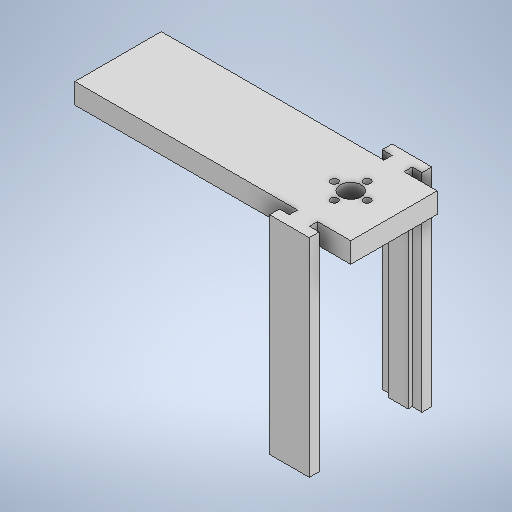
# Autodesk Inventor part: ClawGrip
Saved by Autodesk Inventor 2027 (Build 310192060, 192F)
## iProperties
Created: 2026-06-30
Part Number: ClawGrip
Material: Generic
Document SubType Name: Modeling
Designer: 13129
Density: 1 g/cm^3
Appearance: Default
Author: 13129
Autodesk Inventor part; units mm, degrees
ref_plane "YZ Plane" through (0, 0, 0) normal (1, 0, 0) x (0, 1, 0)
ref_plane "XZ Plane" through (0, 0, 0) normal (0, 1, 0) x (-1, 0, 0)
ref_plane "XY Plane" through (0, 0, 0) normal (0, 0, 1) x (1, 0, 0)
sketch "Sketch1" plane through (0, 0, 0) normal (0, 1, 0) x (-1, 0, 0)
  line L0 (0, 0) -> (42.3, 0)
  line L1 (42.3, 0) -> (42.3, -42.3)
  line L2 (42.3, -42.3) -> (0, -42.3)
  line L3 (0, -42.3) -> (0, 0)
  circle A0 centre (21.15, -21.15) radius 5.15
  circle A1 centre (29.15, -21.15) radius 1.8
  circle A2 centre (21.15, -21.15) radius 8
  circle A3 centre (21.15, -13.15) radius 1.8
  circle A4 centre (13.15, -21.15) radius 1.8
  circle A5 centre (21.15, -29.15) radius 1.8
  point P0 (0, -21.15)
  point P1 (21.15, -42.3)
  dimension "d4" = 16
  dimension "d0" = 42.3
  dimension "d2" = 10.3
  dimension "d3" = 3.6
  dimension "d7" = 360
  constraints: 8 end point, 5 centre point, 4 perpendicular, 3 horizontal alignment, 2 midpoint, 1 coincident, 1 horizontal, 1 vertical alignment, 11 other
  measures "d0" distance of L0.start L0.end
  measures "d2" diameter of A0
  measures "d3" diameter of A1
extrude "Extrusion1" add sketch "Sketch1" along normal blind 10 contours L0 L1 L2 L3 | A1 A2 A5 A4 A3
sketch "Sketch2" plane through (0, 10, 0) normal (0, 1, 0) x (1, 0, 0)
  line L0 (-42.3, 0) -> (0, 0) construction
  circle A0 centre (-13.15, 21.15) radius 1.8 construction
  circle A1 centre (-29.15, 21.15) radius 1.8 construction
  line L1 (-42.3, 0) -> (0, 0) construction
  line L2 (-16.25, 0) -> (-16.25, -3.81)
  line L3 (-16.25, -3.81) -> (-26.05, -3.81)
  line L4 (-26.05, -3.81) -> (-26.05, 0)
  line L5 (-26.05, 0) -> (-16.25, 0)
  line L6 (-13.15, 21.15) -> (-29.15, 21.15)
  line L7 (-42.3, 42.3) -> (0, 42.3) construction
  line L8 (-42.3, 42.3) -> (0, 42.3) construction
  line L9 (-16.25, 42.3) -> (-16.25, 46.11)
  line L10 (-16.25, 46.11) -> (-26.05, 46.11)
  line L11 (-26.05, 46.11) -> (-26.05, 42.3)
  line L12 (-26.05, 42.3) -> (-16.25, 42.3)
  line L13 (-16.25, 46.11) -> (-16.25, 46.31)
  line L14 (-16.25, 46.31) -> (-11.424, 46.31)
  line L15 (-11.424, 46.31) -> (-11.424, 51.136)
  line L16 (-26.05, 46.11) -> (-26.05, 46.31)
  line L17 (-26.05, 46.31) -> (-30.876, 46.31)
  line L18 (-30.876, 46.31) -> (-30.876, 51.136)
  line L19 (-30.876, 51.136) -> (-11.424, 51.136)
  line L20 (-16.25, -3.81) -> (-16.25, -4.01)
  line L21 (-16.25, -4.01) -> (-11.424, -4.01)
  line L22 (-11.424, -4.01) -> (-11.424, -8.836)
  line L23 (-26.05, -3.81) -> (-26.05, -4.01)
  line L24 (-26.05, -4.01) -> (-30.876, -4.01)
  line L25 (-30.876, -4.01) -> (-30.876, -8.836)
  line L26 (-30.876, -8.836) -> (-11.424, -8.836)
  point P0 (-21.15, -3.81)
  point P1 (-21.15, 0)
  point P2 (-21.15, 46.11)
  point P3 (-21.15, 42.3)
  dimension "d11" = 3.81
  dimension "d12" = 9.8
  dimension "d28" = 0.2
  dimension "d29" = 4.826
  dimension "d30" = 4.826
  dimension "d31" = 0.2
  dimension "d32" = 4.826
  dimension "d33" = 4.826
  constraints: 50 end point, 12 symmetric about line, 6 perpendicular, 4 point on line, 2 horizontal, 2 midpoint, 2 vertical, 1 collinear, 1 vertical alignment
  measures "d11" distance of L2.start L2.end
  measures "d12" distance of L2.end L3.end
  measures "d28" distance of L9.end L13.end
  measures "d29" distance of L13.end L14.end
  measures "d30" distance of L14.end L15.end
  measures "d31" distance of L10.end L16.end
  measures "d32" distance of L16.end L17.end
  measures "d33" distance of L17.end L18.end
extrude "Extrusion2" add sketch "Sketch2" against normal blind 10
sketch "Sketch3" plane through (0, 0, 0) normal (0, -1, 0) x (1, 0, 0)
  circle A0 centre (-13.15, -21.15) radius 1.8 construction
  circle A1 centre (-29.15, -21.15) radius 1.8 construction
  line L0 (-13.15, -21.15) -> (-29.15, -21.15)
  line L1 (-16.25, 0) -> (-16.25, 4.01) construction
  line L2 (-11.424, 4.01) -> (-11.424, 8.836) construction
  line L3 (-30.876, 8.836) -> (-30.876, 4.01) construction
  line L4 (-30.876, 4.01) -> (-26.05, 4.01) construction
  line L5 (-26.05, 4.01) -> (-26.05, 0) construction
  line L6 (-16.25, 4.01) -> (-11.424, 4.01)
  line L7 (-11.424, 4.01) -> (-11.424, 8.836)
  line L8 (-11.424, 8.836) -> (-30.876, 8.836)
  line L9 (-30.876, 8.836) -> (-30.876, 4.01)
  line L10 (-30.876, 4.01) -> (-26.05, 4.01)
  line L11 (-26.05, 4.01) -> (-26.05, 2.105)
  line L12 (-26.05, 2.105) -> (-16.25, 2.005)
  line L13 (-16.25, 4.01) -> (-16.25, 2.005)
  line L14 (-16.25, -42.3) -> (-16.25, -46.31) construction
  line L15 (-16.25, -46.31) -> (-11.424, -46.31) construction
  line L16 (-11.424, -46.31) -> (-11.424, -51.136) construction
  line L17 (-11.424, -51.136) -> (-30.876, -51.136) construction
  line L18 (-30.876, -51.136) -> (-30.876, -46.31) construction
  line L19 (-30.876, -46.31) -> (-26.05, -46.31) construction
  line L20 (-26.05, -46.31) -> (-26.05, -42.3) construction
  line L21 (-16.25, -46.31) -> (-11.424, -46.31)
  line L22 (-11.424, -46.31) -> (-11.424, -51.136)
  line L23 (-11.424, -51.136) -> (-30.876, -51.136)
  line L24 (-30.876, -51.136) -> (-30.876, -46.31)
  line L25 (-30.876, -46.31) -> (-26.05, -46.31)
  line L26 (-26.05, -46.31) -> (-26.05, -44.405)
  line L27 (-26.05, -44.405) -> (-16.25, -44.305)
  line L28 (-16.25, -46.31) -> (-16.25, -44.305)
  dimension "d34" = 1.905
  constraints: 48 end point, 6 symmetric about line, 4 collinear, 2 perpendicular, 2 point on line, 1 horizontal, 1 midpoint
  measures "d34" distance of L4.end L11.end
extrude "Extrusion3" add sketch "Sketch3" along normal blind 91.6
sketch "Sketch4" plane through (0, 10, 0) normal (0, 1, 0) x (1, 0, 0)
  line L0 (-42.3, 0) -> (-135.01, 0)
  line L1 (-135.01, 0) -> (-135.01, 42.3)
  line L2 (-135.01, 42.3) -> (-42.3, 42.3)
  line L3 (-42.3, 0) -> (-42.3, 42.3)
  dimension "d17" = 92.71
  constraints: 8 end point, 3 perpendicular, 1 horizontal
  measures "d17" distance of L0.start L0.end
extrude "Extrusion4" add sketch "Sketch4" against normal blind 10
sketch "Sketch5" plane through (0, 0, 0) normal (0, -1, 0) x (1, 0, 0)
  line L0 (-135.01, 0) -> (-135.01, -42.3) construction
  line L1 (-122.31, -36.0725) -> (-51.19, -36.0725)
  line L2 (-51.19, -36.0725) -> (-51.19, -6.2275)
  line L3 (-51.19, -6.2275) -> (-122.31, -6.2275)
  line L4 (-122.31, -6.2275) -> (-122.31, -36.0725)
  point P0 (-135.01, -7.62)
  point P1 (-135.01, -34.68)
  point P2 (-122.31, -21.15)
  point P3 (-135.01, -21.15)
  dimension "d35" = 71.12
  dimension "d36" = 29.845
  dimension "d37" = 12.7
  constraints: 8 end point, 2 midpoint, 2 parallel, 1 horizontal, 1 horizontal alignment, 1 perpendicular
  measures "d35" distance of L3.end L2.end
  measures "d36" distance of L2.end L1.end
  measures "d37" distance between parallel lines of L0 L4
extrude "Extrusion5" cut sketch "Sketch5" against normal blind 5
sketch "Sketch6" plane through (0, 10, 0) normal (0, 1, 0) x (1, 0, 0)
  line L0 (-135.01, 0) -> (-26.05, 0) construction
  line L1 (-30.876, -8.836) -> (-11.424, -8.836) construction
  line L2 (0, 0) -> (0, 42.3) construction
  line L3 (-11.424, 51.136) -> (-30.876, 51.136) construction
  line L4 (-30.876, 51.136) -> (-30.876, 46.31) construction
  line L5 (-26.05, 42.3) -> (-135.01, 42.3) construction
  line L6 (-135.01, 42.3) -> (-135.01, 0) construction
  circle A0 centre (-21.15, 21.15) radius 5.15 construction
  circle A1 centre (-21.15, 21.15) radius 11.43
  line L7 (0, 42.3) -> (0, 0)
  line L8 (0, 0) -> (-11.424, -8.836)
  line L9 (0, 42.3) -> (-11.424, 51.136)
  line L10 (-11.424, 51.136) -> (-30.876, 51.136)
  line L11 (-30.876, 51.136) -> (-30.876, 42.3)
  line L12 (-11.424, -8.836) -> (-30.876, -8.836)
  line L13 (-30.876, -8.836) -> (-30.876, 0)
  line L14 (-30.876, 0) -> (-135.01, 0)
  line L15 (-135.01, 0) -> (-135.01, 42.3)
  line L16 (-135.01, 42.3) -> (-30.876, 42.3)
  dimension "d40" = 22.86
  constraints: 20 end point, 5 collinear, 4 point on line, 1 centre point, 1 coincident, 1 perpendicular
  measures "d40" diameter of A1
extrude "Extrusion6" [suppressed]
chamfer "Chamfer3" [suppressed]
chamfer "Chamfer4" [suppressed]
sketch "Sketch7" plane through (-26.05, 10, -42.3) normal (0, 0, -1) x (-1, 0, 0)
  line L0 (5.08, 0) -> (5.08, 39.5) construction
  line L1 (0, -10) -> (108.96, -10) construction
  circle A0 centre (68.58, 2.7) radius 3.175
  circle A1 centre (55.88, 2.7) radius 3.175
  circle A2 centre (43.18, 2.7) radius 3.175
  circle A3 centre (30.48, 2.7) radius 3.175
  circle A4 centre (17.78, 2.7) radius 3.175
  circle A5 centre (62.23, 15.4) radius 3.175
  circle A6 centre (49.53, 15.4) radius 3.175
  circle A7 centre (36.83, 15.4) radius 3.175
  circle A8 centre (24.13, 15.4) radius 3.175
  circle A9 centre (11.43, 15.4) radius 3.175
  point P0 (101.34, -10)
  point P1 (-26.05, -10)
  dimension "d49" = 6.35
  dimension "d50" = 12.7
  dimension "d51" = 12.7
  dimension "d52" = 12.7
  dimension "d53" = 12.7
  dimension "d54" = 12.7
  dimension "d55" = 12.7
  dimension "d56" = 6.35
  dimension "d57" = 12.7
  dimension "d58" = 12.7
  dimension "d59" = 12.7
  dimension "d60" = 12.7
  dimension "d61" = 6.35
  dimension "d62" = 12.7
  constraints: 10 centre point, 8 equal radius, 8 horizontal alignment
  measures "d49" diameter of A0
  measures "d50" distance of A1.centre A0.centre
  measures "d51" distance of A2.centre A1.centre
  measures "d52" distance of A3.centre A2.centre
  measures "d53" distance of A4.centre A3.centre
  measures "d54" distance from line of L1 A2.centre
  measures "d55" distance from line of L0 A4.centre
  measures "d56" diameter of A5
  measures "d57" distance of A6.centre A5.centre
  measures "d58" distance of A7.centre A6.centre
  measures "d59" distance of A8.centre A7.centre
  measures "d60" distance of A9.centre A8.centre
  measures "d61" distance from line of L0 A9.centre
  measures "d62" vertical distance of A8.centre A3.centre
extrude "Extrusion7" [suppressed]
body "Solid1"
